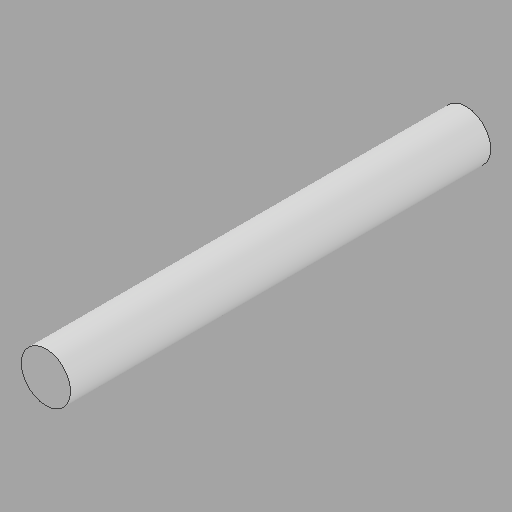
# Autodesk Inventor part: Деталь3
Saved by Autodesk Inventor 2023 (Build 270158000, 158)
## iProperties
Created: 2025-01-12
Part Number: Деталь3
Material: Типовые
Document SubType Name: Modeling
Designer: Ivan
Density: 1 g/cm^3
Appearance: По умолчанию
Author: Ivan
Autodesk Inventor part; units mm, degrees
ref_plane "YZ Plane" through (0, 0, 0) normal (1, 0, 0) x (0, 1, 0)
ref_plane "XZ Plane" through (0, 0, 0) normal (0, 1, 0) x (-1, 0, 0)
sketch "Эскиз1" plane through (0, 0, 0) normal (0, 0, 1) x (1, 0, 0)
  circle A0 centre (0, 0) radius 3
  circle A1 centre (0, 0) radius 5
  constraints: 2 centre point, 4 other
ref_plane "РабПлоскость1" through (-4.125, -3.9693, 51.15) normal (0, 0, 1) x (0.866, 0.5, 0)
extrude "Выдавливание1" add sketch "Эскиз1" along normal up to surface (51.15 mm away) contours A0
